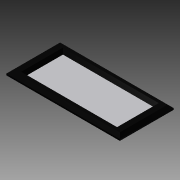
# Autodesk Inventor part: Display
Saved by Autodesk Inventor 2013 SP1 (Build 170176100, 176)
## iProperties
Created: 2013-01-02
Part Number: Display
Material: Kunststoff, undurchsichtig schwarz
Document SubType Name: Modeling
Designer: Sebastian
Density: 1 g/cm^3
Author: Sebastian
Autodesk Inventor part; units mm, degrees
ref_plane "YZ Plane" through (0, 0, 0) normal (1, 0, 0) x (0, 1, 0)
ref_plane "XZ Plane" through (0, 0, 0) normal (0, 1, 0) x (-1, 0, 0)
ref_plane "XY Plane" through (0, 0, 0) normal (0, 0, 1) x (1, 0, 0)
sketch "Skizze1" plane through (0, 0, 0) normal (0, 0, 1) x (1, 0, 0)
  line L0 (-38.4, 18.2) -> (38.4, 18.2)
  line L1 (38.4, 18.2) -> (38.4, -18.2)
  line L2 (38.4, -18.2) -> (-38.4, -18.2)
  line L3 (-38.4, -18.2) -> (-38.4, 18.2)
  line L4 (-38.4, 18.2) -> (38.4, -18.2) construction
  line L5 (38.4, 18.2) -> (-38.4, -18.2) construction
  line L6 (30.4, 12.1) -> (-30.4, 12.1)
  line L7 (-30.4, 12.1) -> (-30.4, -12.1)
  line L8 (-30.4, -12.1) -> (30.4, -12.1)
  line L9 (30.4, -12.1) -> (30.4, 12.1)
  line L10 (30.4, 12.1) -> (-30.4, -12.1) construction
  line L11 (-30.4, 12.1) -> (30.4, -12.1) construction
  point P0 (0, 0)
  dimension "d0" = 76.8
  dimension "d1" = 36.4
  dimension "d2" = 60.8
  dimension "d3" = 24.2
  constraints: 24 end point, 4 midpoint, 4 parallel, 2 horizontal, 2 perpendicular
  measures "d0" distance of L1.end L2.end
  measures "d1" distance of L0.end L1.end
  measures "d2" distance of L8.end L7.end
  measures "d3" distance of L7.end L6.end
extrude "Extrusion1" add sketch "Skizze1" along normal blind 3
sketch "Skizze2" plane through (0, 0, 0) normal (0, 0, 1) x (1, 0, 0)
  line L0 (30.4, 12.1) -> (-30.4, 12.1)
  line L1 (-30.4, 12.1) -> (-30.4, -12.1)
  line L2 (-30.4, -12.1) -> (30.4, -12.1)
  line L3 (30.4, -12.1) -> (30.4, 12.1)
  line L4 (30.4, 12.1) -> (-30.4, -12.1) construction
  line L5 (-30.4, 12.1) -> (30.4, -12.1) construction
  point P0 (0, 0)
  dimension "d6" = 60.8
  dimension "d7" = 24.2
  constraints: 12 end point, 2 midpoint, 2 parallel, 1 horizontal, 1 perpendicular
  measures "d6" distance of L2.end L1.end
  measures "d7" distance of L1.end L0.end
extrude "Extrusion2" add sketch "Skizze2" along normal blind 1 separate body
chamfer "Fase1" distance 2 angle 45 4 edges at (0, 12.1, 3) (-30.4, 0, 3) (0, -12.1, 3) (30.4, 0, 3)
chamfer "Fase2" distance 2 angle 45 4 edges at (38.4, 0, 3) (0, 18.2, 3) (-38.4, 0, 3) (0, -18.2, 3)
